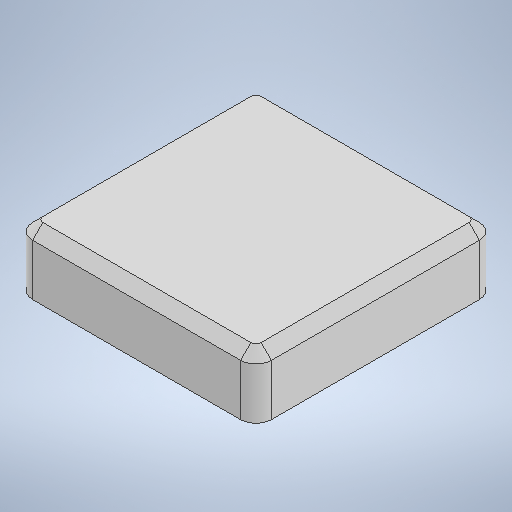
# Autodesk Inventor part: IMU_mount_cover
Saved by Autodesk Inventor 2025.2 (Build 292293000, 293)
## iProperties
Created: 2024-11-14
Part Number: IMU_mount_cover
Material: Generic
Document SubType Name: Modeling
Designer: matss
Density: 1 g/cm^3
Appearance: Default
Author: matss
Autodesk Inventor part; units mm, degrees
ref_plane "YZ Plane" through (0, 0, 0) normal (1, 0, 0) x (0, 1, 0)
ref_plane "XZ Plane" through (0, 0, 0) normal (0, 1, 0) x (-1, 0, 0)
ref_plane "XY Plane" through (0, 0, 0) normal (0, 0, 1) x (1, 0, 0)
sketch "Sketch1" plane through (0, 0, 0) normal (0, 1, 0) x (-1, 0, 0)
  line L0 (20.25, -20.25) -> (-20.25, -20.25)
  line L1 (-20.25, -20.25) -> (-20.25, 20.25)
  line L2 (-20.25, 20.25) -> (20.25, 20.25)
  line L3 (20.25, 20.25) -> (20.25, -20.25)
  line L4 (23.25, 23.25) -> (-23.25, 23.25)
  line L5 (-23.25, 23.25) -> (-23.25, -23.25)
  line L6 (-23.25, -23.25) -> (23.25, -23.25)
  line L7 (23.25, -23.25) -> (23.25, 23.25)
  point P0 (0, 0)
  point P1 (20.25, 0)
  point P2 (0, -20.25)
  point P3 (23.25, 0)
  point P4 (0, -23.25)
  dimension "d0" = 40.5
  dimension "d1" = 40.5
  dimension "d2" = 46.5
  dimension "d3" = 46.5
  constraints: 16 end point, 4 midpoint, 4 parallel, 2 horizontal, 2 horizontal alignment, 2 perpendicular, 2 vertical alignment
  measures "d0" distance of L0.start L0.end
  measures "d1" distance of L2.end L0.start
  measures "d2" distance of L6.end L4.start
  measures "d3" distance of L5.end L6.end
extrude "Extrusion1" add sketch "Sketch1" along normal blind 10
fillet "Fillet1" radius 3 8 edges at (-23.25, 5, 23.25) (23.25, 5, 23.25) (23.25, 5, -23.25) (-23.25, 5, -23.25) (-20.25, 5, -20.25) (-20.25, 5, 20.25) (20.25, 5, 20.25) (20.25, 5, -20.25)
ref_plane "Arbeitsebene3" through (-17.25, 0, -20.25) normal (1, 0, 0) x (0, 1, 0)
sketch "Skizze10" plane through (0, 10, 0) normal (0, 1, 0) x (1, 0, 0)
  line L0 (20.25, 23.25) -> (-20.25, 23.25) projected
  arc A0 (-20.25, 23.25) -> (-23.25, 20.25) centre (-20.25, 20.25) ccw projected
  line L1 (-23.25, 20.25) -> (-23.25, -20.25) projected
  arc A1 (-23.25, -20.25) -> (-20.25, -23.25) centre (-20.25, -20.25) ccw projected
  line L2 (-20.25, -23.25) -> (20.25, -23.25) projected
  arc A2 (20.25, -23.25) -> (23.25, -20.25) centre (20.25, -20.25) ccw projected
  line L3 (23.25, -20.25) -> (23.25, 20.25) projected
  arc A3 (23.25, 20.25) -> (20.25, 23.25) centre (20.25, 20.25) ccw projected
  line L4 (-20.25, 23.25) -> (20.25, 23.25)
  line L5 (23.25, 20.25) -> (23.25, -20.25)
  line L6 (20.25, -23.25) -> (-20.25, -23.25)
  line L7 (-23.25, -20.25) -> (-23.25, 20.25)
  arc A4 (-20.25, 23.25) -> (-23.25, 20.25) centre (-20.25, 20.25) ccw
  arc A5 (23.25, 20.25) -> (20.25, 23.25) centre (20.25, 20.25) ccw
  arc A6 (20.25, -23.25) -> (23.25, -20.25) centre (20.25, -20.25) ccw
  arc A7 (-23.25, -20.25) -> (-20.25, -23.25) centre (-20.25, -20.25) ccw
  line L8 (-20.25, -23.25) -> (20.25, -23.25)
  point P0 (0, 0)
  constraints: 11 point on circle, 10 end point, 4 centre point, 4 coincident, 2 collinear, 1 horizontal, 1 point on line
extrude "Extrusion6" add sketch "Skizze10" along normal blind 2
sketch "Skizze9" plane through (-17.25, 0, -20.25) normal (1, 0, 0) x (0, 1, 0)
  line L0 (10, 0) -> (0, 0) construction
  line L1 (6.2, 0) -> (6.2, 0.8787) construction
  arc A0 (3.3, 0) -> (1.3, 0) centre (2.3, 0) ccw
  line L2 (3.3, 0) -> (1.3, 0)
  line L3 (10, 3) -> (10, 37.5) projected
  line L4 (6.2, 20.25) -> (0, 20.25)
  line L5 (6.2, 40.5) -> (0, 40.5) construction
  arc A1 (1.3, 40.5) -> (3.3, 40.5) centre (2.3, 40.5) ccw
  line L6 (3.3, 40.5) -> (1.3, 40.5)
  point P0 (4.6, 0)
  point P1 (6.2, 3)
  point P2 (6.2, 15.294)
  dimension "d51" = 1.6
  dimension "d52" = 2.3
  dimension "d53" = 1
  constraints: 8 end point, 6 point on line, 4 point on circle, 4 symmetric about line, 2 centre point, 1 coincident, 1 collinear, 1 horizontal, 4 other
  measures "d51" distance from line of L1 point (4.6, 0)
  measures "d52" distance of point (4.6, 0) point (2.3, 0)
  measures "d53" distance of point (2.3, 0) L2.end
extrude "Extrusion5" add sketch "Skizze9" along normal blind 37.5 and the other way blind 3
chamfer "Fasen1" distance 2 angle 45 8 edges at (-23.25, 12, 0) (-22.3713, 12, 22.3713) (0, 12, 23.25) (22.3713, 12, 22.3713) (23.25, 12, 0) (22.3713, 12, -22.3713) (0, 12, -23.25) (-22.3713, 12, -22.3713)
body "Solid1"
